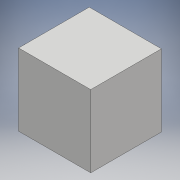
# Autodesk Inventor part: Part1
Saved by Autodesk Inventor 2017 (Build 210142000, 142)
## iProperties
Created: 2020-06-12
Part Number: Part1
Material: Generic
Document SubType Name: Modeling
Designer: DML
Density: 1 g/cm^3
Appearance: Default
Author: DML
Autodesk Inventor part; units mm, degrees
ref_plane "YZ Plane" through (0, 0, 0) normal (1, 0, 0) x (0, 1, 0)
ref_plane "XZ Plane" through (0, 0, 0) normal (0, 1, 0) x (-1, 0, 0)
ref_plane "XY Plane" through (0, 0, 0) normal (0, 0, 1) x (1, 0, 0)
sketch "Sketch2" plane through (0, 0, 0) normal (0, 1, 0) x (-1, 0, 0)
  line L0 (0, 0) -> (50, 0)
  line L1 (50, 0) -> (50, -50)
  line L2 (50, -50) -> (0, -50)
  line L3 (0, -50) -> (0, 0)
  dimension "d0" = 50
  dimension "d1" = 50
  constraints: 8 end point, 2 parallel, 1 horizontal, 1 perpendicular
  measures "d0" distance of L1.end L2.end
  measures "d1" distance of L0.end L1.end
extrude "Extrusion1" add sketch "Sketch2" along normal blind 4
sketch "Sketch3" plane through (0, 4, 0) normal (0, 1, 0) x (1, 0, 0)
  line L0 (0, 0) -> (0, 50) projected
  line L1 (-50.0118, 0) -> (0, 0)
  line L2 (0, 0) -> (0, 50)
  line L3 (0, 50) -> (-50.0118, 50)
  line L4 (-50.0118, 50) -> (-50.0118, 0)
  line L5 (-48.0118, 2) -> (-2, 2)
  line L6 (-2, 2) -> (-2, 48)
  line L7 (-2, 48) -> (-48.0118, 48)
  line L8 (-48.0118, 48) -> (-48.0118, 2)
  dimension "d4" = 2
  constraints: 16 end point, 4 parallel, 2 perpendicular, 1 horizontal, 3 other
  measures "d4" distance between parallel lines of L4 L8
extrude "Extrusion2" add sketch "Sketch3" along normal blind 45
body "Solid1"
